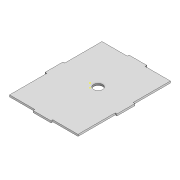
# Autodesk Inventor part: 본체 밑판 레이저 커터
Saved by Autodesk Inventor 2020 (Build 240168000, 168)
## iProperties
Created: 2022-08-24
Part Number: 본체 밑판 레이저 커터
Material: 일반
Document SubType Name: Modeling
Designer: 박연호
Density: 1 g/cm^3
Appearance: 기본값
Author: 박연호
Autodesk Inventor part; units mm, degrees
ref_plane "YZ Plane" through (0, 0, 0) normal (1, 0, 0) x (0, 1, 0)
ref_plane "XZ Plane" through (0, 0, 0) normal (0, 1, 0) x (-1, 0, 0)
ref_plane "XY Plane" through (0, 0, 0) normal (0, 0, 1) x (1, 0, 0)
sketch "스케치1" plane through (0, 0, 0) normal (0, 1, 0) x (-1, 0, 0)
  line L0 (60, 80) -> (-60, 80)
  line L1 (-60, 80) -> (-60, -80)
  line L2 (-60, -80) -> (60, -80)
  line L3 (60, -80) -> (60, 80)
  line L4 (60, 80) -> (-60, -80) construction
  line L5 (-60, 80) -> (60, -80) construction
  point P0 (0, 0)
  dimension "d0" = 120
  dimension "d1" = 160
  constraints: 12 end point, 2 midpoint, 2 parallel, 1 horizontal, 1 perpendicular
  measures "d0" distance of L0.start L0.end
  measures "d1" distance of L0.end L1.end
extrude "돌출1" add sketch "스케치1" along normal blind 60
sketch "스케치2" plane through (0, 60, 0) normal (0, 1, 0) x (1, 0, 0)
  line L0 (60, -80) -> (60, 80) projected
  line L1 (60, 80) -> (-60, 80) projected
  line L2 (55, 102.1646) -> (-55, 102.1646)
  line L3 (-55, 102.1646) -> (-55, -89.711)
  line L4 (-55, -89.711) -> (55, -89.711)
  line L5 (55, -89.711) -> (55, 102.1646)
  line L6 (-60, 80) -> (-60, -80) projected
  point P0 (0, 0)
  point P1 (55, 80)
  point P2 (-55, 80)
  dimension "d6" = 5
  dimension "d7" = 5
  constraints: 8 end point, 2 parallel, 1 horizontal, 1 perpendicular
  measures "d6" distance between parallel lines of L5 L0
  measures "d7" distance between parallel lines of L6 L3
extrude "돌출2" cut sketch "스케치2" against normal blind 40 contours L5 L4 L3 L1
sketch "스케치12" plane through (60, 0, -80) normal (0, 0, -1) x (-1, 0, 0)
  line L0 (-34.8463, 10) -> (156.2634, 10)
  line L1 (156.2634, 10) -> (156.2634, -36.9465)
  line L2 (156.2634, -36.9465) -> (-34.8463, -36.9465)
  line L3 (-34.8463, -36.9465) -> (-34.8463, 10)
  line L4 (0, 0) -> (120, 0) projected
  point P0 (60, 0)
  dimension "d85" = 10
  constraints: 8 end point, 2 parallel, 1 horizontal, 1 perpendicular
  measures "d85" distance between parallel lines of L4 L0
extrude "돌출10" cut sketch "스케치12" against normal through all
sketch "스케치13" plane through (-55, 20, 80) normal (0, 0, 1) x (1, 0, 0)
  line L0 (0, 40) -> (0, 0) projected
  line L1 (0, 0) -> (110, 0) projected
  line L2 (0, 40) -> (110, 40)
  line L3 (110, 40) -> (110, 0)
  line L4 (110, 0) -> (0, 0)
  line L5 (0, 0) -> (0, 40)
  point P0 (55, -20)
  constraints: 8 end point, 2 parallel, 1 horizontal, 1 perpendicular
extrude "돌출11" add sketch "스케치13" against normal blind 5
sketch "스케치14" plane through (55, 20, -80) normal (0, 0, -1) x (-1, 0, 0)
  line L0 (0, 0) -> (0, 40) projected
  line L1 (110, 0) -> (0, 0) projected
  line L2 (0, 40) -> (110, 40)
  line L3 (110, 40) -> (110, 0)
  line L4 (110, 0) -> (0, 0)
  line L5 (0, 0) -> (0, 40)
  point P0 (55, -20)
  constraints: 8 end point, 2 parallel, 1 horizontal, 1 perpendicular
extrude "돌출12" add sketch "스케치14" against normal blind 5
sketch "스케치15" plane through (60, 60, -80) normal (0, 0, -1) x (-1, 0, 0)
  point P0 (60, -60)
sketch "스케치16" plane through (60, 60, -80) normal (0, 0, -1) x (-1, 0, 0)
  point P0 (60, -60)
sketch "스케치21" plane through (0, 20, 0) normal (0, 1, 0) x (1, 0, 0)
  circle A0 centre (5.4243, 8.1678) radius 7.5
  line L0 (-49.3888, 17.2731) -> (-9.3888, 17.2731)
  line L1 (-9.3888, 17.2731) -> (-9.3888, 67.2731)
  line L2 (-9.3888, 67.2731) -> (-49.3888, 67.2731)
  line L3 (-49.3888, 67.2731) -> (-49.3888, 17.2731)
  point P0 (0, 0)
  dimension "d117" = 15
  dimension "d118" = 50
  dimension "d119" = 40
  constraints: 8 end point, 2 parallel, 1 centre point, 1 horizontal, 1 perpendicular
  measures "d117" diameter of A0
  measures "d118" distance of L2.end L0.start
  measures "d119" distance of L1.end L2.end
extrude "돌출15" cut sketch "스케치21" against normal through all contours A0
sketch "스케치24" plane through (0, 60, 0) normal (0, 1, 0) x (1, 0, 0)
  line L0 (-60, 80) -> (-60, -80) projected
  line L1 (60, 80) -> (-60, 80) projected
  line L2 (-60, -80) -> (60, -80)
  line L3 (60, -80) -> (60, 80)
  line L4 (60, 80) -> (-60, 80)
  line L5 (-60, 80) -> (-60, -80)
  point P0 (0, 0)
  constraints: 8 end point, 2 parallel, 1 horizontal, 1 perpendicular
extrude "돌출17" cut sketch "스케치24" against normal blind 40
sketch "스케치25" plane through (60, 20, -80) normal (0, 0, -1) x (-1, 0, 0)
  point P0 (60, -20)
sketch "스케치26" plane through (0, 20, 0) normal (0, 1, 0) x (1, 0, 0)
  point P0 (0, 0)
sketch "스케치27" plane through (0, 20, 0) normal (0, 1, 0) x (1, 0, 0)
  line L0 (-60, -80) -> (-60, 80) projected
  line L1 (60, 80) -> (60, -80) projected
  line L2 (-60, -80) -> (60, -80)
  line L3 (60, -80) -> (60, 80)
  line L4 (60, 80) -> (-60, 80)
  line L5 (-60, 80) -> (-60, -80)
  point P0 (0, 0)
  point P1 (60, -80)
  constraints: 8 end point, 2 parallel, 1 horizontal, 1 perpendicular
extrude "돌출18" cut sketch "스케치27" against normal blind 7
sketch "스케치30" plane through (0, 13, 0) normal (0, 1, 0) x (1, 0, 0)
  point P0 (0, 0)
sketch "스케치31" plane through (0, 13, 0) normal (0, 1, 0) x (1, 0, 0)
  line L0 (-60, -80) -> (-60, 80) projected
  line L1 (60, -80) -> (-60, -80) projected
  line L2 (60, 80) -> (60, -80) projected
  line L3 (-60, 80) -> (60, 80) projected
  line L4 (57, 77) -> (57, -77)
  line L5 (57, -77) -> (-57, -77)
  line L6 (-57, -77) -> (-57, 77)
  line L7 (-57, 77) -> (57, 77)
  point P0 (0, 0)
  dimension "d160" = 3
  constraints: 8 end point, 3 other
  measures "d160" distance between parallel lines of L3 L7
extrude "돌출21" cut sketch "스케치31" against normal through all
sketch "스케치32" plane through (0, 13, 0) normal (0, 1, 0) x (1, 0, 0)
  line L0 (-15, 68.5163) -> (15, 68.5163)
  line L1 (15, 68.5163) -> (15, 80)
  line L2 (15, 80) -> (-15, 80)
  line L3 (-15, 80) -> (-15, 68.5163)
  line L4 (57, 77) -> (-57, 77) projected
  line L5 (-57, 77) -> (-57, -77) projected
  line L6 (-57, 0) -> (57, 0)
  line L7 (-15, -68.5163) -> (15, -68.5163)
  line L8 (15, -68.5163) -> (15, -80)
  line L9 (15, -80) -> (-15, -80)
  line L10 (-15, -80) -> (-15, -68.5163)
  line L11 (-57, -77) -> (57, -77) projected
  point P0 (0, 0)
  point P1 (-15, 77)
  point P2 (15, 77)
  point P3 (15, -77)
  point P4 (-15, -77)
  dimension "d163" = 3
  dimension "d164" = 42
  dimension "d165" = 30
  constraints: 18 end point, 4 symmetric about line, 2 horizontal, 2 parallel, 1 midpoint, 1 perpendicular
  measures "d163" distance between parallel lines of L4 L2
  measures "d164" distance between parallel lines of L5 L3
  measures "d165" distance of L1.end L2.end
extrude "돌출22" add sketch "스케치32" against normal blind 3 contours L11 L8 L9 L10 | L3 L2 L1 L4
sketch "스케치33" plane through (0, 13, 0) normal (0, 1, 0) x (1, 0, 0)
  line L0 (44.1532, -15) -> (60, -15)
  line L1 (60, -15) -> (60, 15)
  line L2 (60, 15) -> (44.1532, 15)
  line L3 (44.1532, 15) -> (44.1532, -15)
  line L4 (57, -77) -> (57, 77) projected
  line L5 (57, 77) -> (15, 77) projected
  line L6 (-57, 77) -> (-57, -77) projected
  line L7 (-15, 80) -> (15, 80) projected
  line L8 (0, 80) -> (0, -80)
  line L9 (15, -80) -> (-15, -80) projected
  line L10 (-44.1532, -15) -> (-60, -15)
  line L11 (-60, -15) -> (-60, 15)
  line L12 (-60, 15) -> (-44.1532, 15)
  line L13 (-44.1532, 15) -> (-44.1532, -15)
  point P0 (0, 0)
  point P1 (57, 15)
  point P2 (57, -15)
  point P3 (-57, -15)
  point P4 (-57, 15)
  dimension "d168" = 3
  dimension "d169" = 30
  dimension "d170" = 62
  constraints: 18 end point, 4 symmetric about line, 2 midpoint, 2 parallel, 1 horizontal, 1 perpendicular
  measures "d168" distance between parallel lines of L1 L4
  measures "d169" distance of L0.end L1.end
  measures "d170" distance between parallel lines of L5 L2
extrude "돌출23" add sketch "스케치33" against normal blind 3 contours L4 L2 L1 L0 | L6 L10 L11 L12
sketch "스케치34" plane through (0, 13, 0) normal (0, 1, 0) x (1, 0, 0)
  point P0 (0, 0)
sketch "스케치35" plane through (0, 13, 0) normal (0, 1, 0) x (1, 0, 0)
  point P0 (0, 0)
